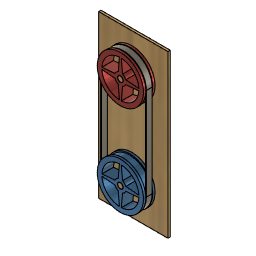
1 - Simple Pulley (Autodesk Fusion 360 design; units mm, degrees)
Autodesk Fusion 360 part; units mm, degrees
sketch "Sketch1" plane through (0, 0, 0) normal (0, 1, 0) x (1, 0, 0)
  circle A0 centre (0, 0) radius 25.4
  line L0 (-5.902, 2.3429) -> (-20.3281, 1.0808)
  line L1 (-5.902, 2.3429) -> (8.5793, 2.3429) construction
  line L2 (2.5, 0) -> (20, 0)
  line L3 (-5.902, -2.3429) -> (-20.3281, -1.0808)
  line L4 (2.3429, -5.902) -> (1.0808, -20.3281)
  line L5 (-2.3429, -5.902) -> (-1.0808, -20.3281)
  line L6 (5.902, 2.3429) -> (20.3281, 1.0808)
  line L7 (5.902, -2.3429) -> (20.3281, -1.0808)
  line L8 (-2.3429, 5.902) -> (-1.0808, 20.3281)
  line L9 (2.3429, 5.902) -> (1.0808, 20.3281)
  arc A1 (-20.2911, -1.0841) -> (-1.0841, -20.2911) centre (0, 0) ccw
  arc A2 (1.0841, -20.2911) -> (20.2911, -1.0841) centre (0, 0) ccw
  arc A3 (5.902, 2.3429) -> (2.3429, 5.902) centre (0, 0) ccw
  arc A4 (-2.3429, 5.902) -> (-5.902, 2.3429) centre (0, 0) ccw
  arc A5 (-5.902, -2.3429) -> (-2.3429, -5.902) centre (0, 0) ccw
  arc A6 (2.3429, -5.902) -> (5.902, -2.3429) centre (0, 0) ccw
  arc A7 (20.2911, 1.0841) -> (1.0841, 20.2911) centre (0, 0) ccw
  arc A8 (-1.0841, 20.2911) -> (-20.2911, 1.0841) centre (0, 0) ccw
  dimension "d1" = 50.8
  dimension "d3" = 12.7
  dimension "d4" = 175
  dimension "d6" = 360
  constraint coincident A0.centre A1.centre
  constraint concentric A0 A3
  constraint horizontal L1
  constraint symmetric L0.start L2 L3.start
  constraint symmetric L0.end L2 L3.end
  constraint concentric A0 A1
  constraint coincident L0 A8.end
  constraint coincident L3 A1.start
  constraint coincident L5 A1.end
  constraint coincident L4 A2.start
  constraint concentric A1 A2
  constraint coincident L7 A2.end
  constraint coincident L6 A7.start
  constraint concentric A2 A7
  constraint concentric A3 A5
  constraint concentric A3 A4
  constraint concentric A5 A6
  constraint coincident L9 A7.end
  constraint coincident L8 A8.start
  constraint concentric A7 A8
  measures "d1" diameter of A0
  measures "d3" diameter of A3
  measures "d4" angle of L0 L1
extrude "Extrude1" add sketch "Sketch1" along normal blind 12.7 makes body 1
sketch "Sketch2" plane through (0, 0, 0) normal (0, -1, 0) x (1, 0, 0)
  line L0 (-2.3429, -5.902) -> (-1.0841, -20.2911)
  arc A0 (-20.2911, -1.0841) -> (-1.0841, -20.2911) centre (0, 0) ccw
  line L1 (-20.2911, -1.0841) -> (-5.902, -2.3429)
  arc A1 (-5.902, -2.3429) -> (-2.3429, -5.902) centre (0, 0) ccw
  line L2 (5.902, -2.3429) -> (20.2911, -1.0841)
  arc A2 (1.0841, -20.2911) -> (20.2911, -1.0841) centre (0, 0) ccw
  line L3 (1.0841, -20.2911) -> (2.3429, -5.902)
  arc A3 (2.3429, -5.902) -> (5.902, -2.3429) centre (0, 0) ccw
  arc A4 (20.2911, 1.0841) -> (1.0841, 20.2911) centre (0, 0) ccw
  line L4 (20.2911, 1.0841) -> (5.902, 2.3429)
  arc A5 (5.902, 2.3429) -> (2.3429, 5.902) centre (0, 0) ccw
  line L5 (2.3429, 5.902) -> (1.0841, 20.2911)
  arc A6 (-1.0841, 20.2911) -> (-20.2911, 1.0841) centre (0, 0) ccw
  line L6 (-1.0841, 20.2911) -> (-2.3429, 5.902)
  arc A7 (-2.3429, 5.902) -> (-5.902, 2.3429) centre (0, 0) ccw
  line L7 (-5.902, 2.3429) -> (-20.2911, 1.0841)
  circle A8 centre (0, 0) radius 25.4
  circle A9 centre (0, 0) radius 25.4
  circle A10 centre (0, 0) radius 24.13
  dimension "d9" = -1.27
extrude "Extrude2" cut sketch "Sketch2" against normal blind 7.62 from surface at -2.54 contours A8 A9 bodies 1
ref_plane "WorkPlane1" through (0, 0, -50.8) normal (0, 0, 1) x (1, 0, 0)
mirror "Mirror1" about plane through (0, 0, -50.8) normal (0, 0, 1) of bodies 1 makes body 2
ref_plane "WorkPlane2" through (0, 6.35, 0) normal (0, 1, 0) x (0, 0, 1)
sketch "Sketch3" plane through (0, 6.35, 0) normal (0, 1, 0) x (1, 0, 0)
  circle A0 centre (0, 0) radius 24.13
  circle A1 centre (0, 101.6) radius 24.13
  line L0 (0, 0) -> (-24.13, 0)
  line L1 (-24.13, 0) -> (-24.13, 101.6)
  line L2 (0, -20) -> (0, -2.5)
  line L3 (24.13, 0) -> (24.13, 101.6)
  arc A2 (-24.13, 0) -> (24.13, 0) centre (0, 0) ccw
  arc A3 (24.13, 101.6) -> (-24.13, 101.6) centre (0, 101.6) ccw
  arc A4 (-25.146, 0) -> (25.146, 0) centre (0, 0) ccw
  line L4 (25.146, 0) -> (25.146, 101.6)
  arc A5 (25.146, 101.6) -> (-25.146, 101.6) centre (0, 101.6) ccw
  line L5 (-25.146, 0) -> (-25.146, 101.6)
  dimension "d17" = 101.6
  dimension "d18" = -1.016
  constraint coincident A0.centre L0.start
  constraint coincident A0 L0.end
  constraint horizontal L0
  constraint perpendicular L0 L1
  constraint symmetric L0.end L2 L3.start
  constraint symmetric L1.end L2 L3.end
  constraint tangent L3 A2
  constraint tangent L1 A3
  measures "d17" distance of L0.end L1.end
extrude "Extrude3" add sketch "Sketch3" along normal mid plane 6.35 separate body makes body 3
copy_body "Body->Comp1" bodies 3 removing the originals makes body 4 in component "Belt"
copy_body "Body->Comp2" bodies 1 removing the originals makes body 5 in component "Wheel1"
copy_body "Body->Comp3" bodies 2 removing the originals makes body 6 in component "Wheel2"
sketch "Sketch4" plane through (0, 0, 0) normal (0, -1, 0) x (1, 0, 0)
  line L0 (-2.3429, -5.902) -> (-1.0841, -20.2911)
  arc A0 (-20.2911, -1.0841) -> (-1.0841, -20.2911) centre (0, 0) ccw
  line L1 (-20.2911, -1.0841) -> (-5.902, -2.3429)
  arc A1 (-5.902, -2.3429) -> (-2.3429, -5.902) centre (0, 0) ccw
  line L2 (5.902, -2.3429) -> (20.2911, -1.0841)
  arc A2 (1.0841, -20.2911) -> (20.2911, -1.0841) centre (0, 0) ccw
  line L3 (1.0841, -20.2911) -> (2.3429, -5.902)
  arc A3 (2.3429, -5.902) -> (5.902, -2.3429) centre (0, 0) ccw
  arc A4 (20.2911, 1.0841) -> (1.0841, 20.2911) centre (0, 0) ccw
  line L4 (20.2911, 1.0841) -> (5.902, 2.3429)
  arc A5 (5.902, 2.3429) -> (2.3429, 5.902) centre (0, 0) ccw
  line L5 (2.3429, 5.902) -> (1.0841, 20.2911)
  arc A6 (-1.0841, 20.2911) -> (-20.2911, 1.0841) centre (0, 0) ccw
  line L6 (-1.0841, 20.2911) -> (-2.3429, 5.902)
  arc A7 (-2.3429, 5.902) -> (-5.902, 2.3429) centre (0, 0) ccw
  line L7 (-5.902, 2.3429) -> (-20.2911, 1.0841)
  circle A8 centre (0, 0) radius 25.4
  circle A9 centre (0, 0) radius 3.175
  line L8 (0.4291, -50.8) -> (12.4447, -50.8)
  circle A10 centre (0, -101.6) radius 3.175
  dimension "d21" = 6.35
  constraint coincident A0.centre A1.centre
  constraint symmetric A9 L8 A10
  measures "d21" diameter of A9
extrude "Extrude1'" cut sketch "Sketch4" against normal up to surface (12.7 mm away) contours A9 | A10 bodies 5 in component "Wheel1"
extrude "Extrude1''" cut sketch "Sketch4" against normal up to surface (12.7 mm away) contours A9 | A10 bodies 6 in component "Wheel2"
ref_plane "WorkPlane3" through (0, 13.97, 0) normal (0, 1, 0) x (1, 0, 0)
sketch "Sketch5" plane through (0, 13.97, 0) normal (0, 1, 0) x (1, 0, 0)
  line L0 (38.1, -38.1) -> (-38.1, -38.1)
  line L1 (-38.1, -38.1) -> (-38.1, 139.7)
  line L2 (-38.1, 139.7) -> (38.1, 139.7)
  line L3 (38.1, 139.7) -> (38.1, -38.1)
  constraint horizontal L0
  constraint vertical L1
  constraint horizontal L2
  constraint vertical L3
extrude "Extrude4" add sketch "Sketch5" along normal blind 2.54 separate body makes body 7
sketch "Sketch6" plane through (0, 13.97, 0) normal (0, -1, 0) x (1, 0, 0)
  line L0 (-38.1, -139.7) -> (38.1, -139.7)
  line L1 (38.1, -139.7) -> (38.1, 38.1)
  line L2 (38.1, 38.1) -> (-38.1, 38.1)
  line L3 (-38.1, 38.1) -> (-38.1, -139.7)
  circle A0 centre (0, 0) radius 2.8575
  line L4 (0.4291, -50.8) -> (12.4447, -50.8)
  circle A1 centre (0, -101.6) radius 2.8575
  dimension "d29" = 5.715
  constraint coincident A0.centre origin
  constraint symmetric A0 L4 A1
  measures "d29" diameter of A0
extrude "Extrude5" add sketch "Sketch6" along normal blind 14.224 contours A0 | A1 bodies 7
copy_body "Body->Comp4" bodies 7 removing the originals makes body 8 in component "Backboard"
component "Belt" placed x (1, 0, 0) y (0, 1, 0) z (0, 0, 1) at (0, 0, 0)
component "Wheel1" placed x (1, 0, 0) y (0, 1, 0) z (0, 0, 1) at (0, -0.254, 0)
component "Wheel2" placed x (1, 0, 0) y (0, 1, 0) z (0, 0, 1) at (0, -0.254, 0)
component "Backboard" placed x (1, 0, 0) y (0, 1, 0) z (0, 0, 1) at (0, 0, 0)
named bodies: "Wheel1", "Wheel2", "Belt"
